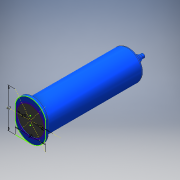
# Autodesk Inventor part: Larger Syringe
Saved by Autodesk Inventor 2016 (Build 200138000, 138)
## iProperties
Created: 2016-05-08
Part Number: Larger Syringe
Material: Generic
Document SubType Name: Modeling
Designer: Kenneth Daniel
Density: 1 g/cm^3
Appearance: Default
Author: Kenneth Daniel
Autodesk Inventor part; units mm, degrees
ref_plane "YZ Plane" through (0, 0, 0) normal (1, 0, 0) x (0, 1, 0)
ref_plane "XZ Plane" through (0, 0, 0) normal (0, 1, 0) x (-1, 0, 0)
ref_plane "XY Plane" through (0, 0, 0) normal (0, 0, 1) x (1, 0, 0)
sketch "Sketch1" plane through (0, 0, 0) normal (0, 1, 0) x (-1, 0, 0)
  circle A0 centre (0, 0) radius 16.5
  line L0 (0, -23.5) -> (18, -23.5)
  line L1 (18, -9.261) -> (18, 9.261)
  line L2 (-18, 9.261) -> (-18, -9.261)
  line L3 (-18, -23.5) -> (18, 23.5) construction
  line L4 (18, -23.5) -> (-18, 23.5) construction
  arc A1 (18, 9.261) -> (-18, 9.261) centre (0, 5.0033) ccw
  line L5 (28.3506, 0) -> (-36.241, 0) construction
  arc A2 (-18, -9.261) -> (18, -9.261) centre (0, -5.0033) ccw
  circle A3 centre (0, 0) radius 17.5
  dimension "d0" = 33
  dimension "d1" = 36
  dimension "d2" = 47
  dimension "d3" = 1
  constraints: 12 end point, 5 point on circle, 4 centre point, 3 symmetric about line, 2 horizontal, 2 midpoint, 1 coincident, 1 parallel, 1 perpendicular, 1 other
  measures "d0" diameter of A0
  measures "d1" distance of L3.start L0.end
  measures "d2" distance of L3.end L0.end
  measures "d3" radial gap between concentric circles of A0 A3
extrude "Extrusion1" add sketch "Sketch1" along normal blind 115 contours A3
extrude "Extrusion2" add sketch "Sketch1" along normal blind 3
sketch "Sketch2" plane through (0, 0, 0) normal (0, 0, 1) x (1, 0, 0)
  line L0 (16.5, 3) -> (16.5, 115) projected
  line L1 (16.5, 115) -> (11, 115)
  line L2 (17.5, 115) -> (-17.5, 115) projected
  line L3 (11, 115) -> (6.2224, 118.6297)
  line L4 (6.2224, 118.6297) -> (3.2708, 127.1319)
  line L5 (3.2708, 127.1319) -> (4.2154, 127.4599)
  line L6 (4.2154, 127.4599) -> (9.99, 118.6297)
  line L7 (17.5, 115) -> (16.6596, 116.8149)
  line L8 (16.6596, 116.8149) -> (9.99, 118.6297)
  line L9 (3.2708, 127.1319) -> (1.9591, 130.9102)
  line L10 (1.9591, 130.9102) -> (2.3904, 131.1923)
  line L11 (2.3904, 131.1923) -> (4.2154, 127.4599)
  line L12 (1.9591, 130.9102) -> (1.9591, 133.9102)
  line L13 (1.9591, 133.9102) -> (2.3904, 133.9102)
  line L14 (2.3904, 133.9102) -> (2.3904, 131.1923)
  line L15 (0, -26.782) -> (0, 160.6923) projected
  point P0 (0, 0)
  dimension "d8" = 5.5
  dimension "d9" = 6
  dimension "d10" = 9
  dimension "d11" = 1
  dimension "d12" = 2
  dimension "d13" = 3
  constraints: 26 end point, 4 perpendicular, 2 point on line, 1 vertical
  measures "d8" distance of L1.start L1.end
  measures "d9" distance of L1.end L3.end
  measures "d10" distance of L3.end L4.end
  measures "d11" distance of L4.end L5.end
  measures "d12" distance of L2.start L7.end
  measures "d13" distance of L9.end L12.end
revolve "Revolution1" add sketch "Sketch2" angle 360 about axis through (0, -10, 0) along (0, 1, 0)
extrude "Extrusion3" cut sketch "Sketch1" along normal blind 1 contours A0
body "Solid1"
